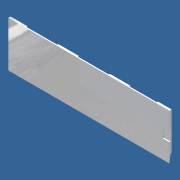
# Autodesk Inventor part: bottom panel left
Saved by Autodesk Inventor 2012 (Build 160160000, 160)
## iProperties
Created: 2012-02-06
Part Number: bottom panel left
Material: Default
Document SubType Name: Modeling
Designer: Allison Garza
Density: 1 g/cm^3
Author: Allison Garza
Autodesk Inventor part; units mm, degrees
ref_plane "YZ Plane" through (0, 0, 0) normal (1, 0, 0) x (0, 1, 0)
ref_plane "XZ Plane" through (0, 0, 0) normal (0, 1, 0) x (-1, 0, 0)
ref_plane "XY Plane" through (0, 0, 0) normal (0, 0, 1) x (1, 0, 0)
sketch "Sketch1" plane through (0, 0, 0) normal (0, 0, 1) x (1, 0, 0)
  line L0 (-37.1429, 20.9244) -> (432.7571, 20.9244)
  line L1 (432.7571, 20.9244) -> (432.7571, -112.4256)
  line L2 (432.7571, -112.4256) -> (-37.1429, -112.4256)
  line L3 (-37.1429, -112.4256) -> (-37.1429, 20.9244)
  point P0 (0, 0)
  dimension "d0" = 469.9
  dimension "d1" = 133.35
  constraints: 8 end point, 2 parallel, 1 horizontal, 1 perpendicular
  measures "d0" distance of L0.start L0.end
  measures "d1" distance of L2.end L0.start
extrude "Extrusion1" add sketch "Sketch1" along normal blind 3.175
sketch "Sketch2" plane through (432.7571, -112.4256, 0) normal (1, 0, 0) x (0, 0, -1)
  line L0 (0, 133.35) -> (0, 0) projected
  line L1 (-3.175, 133.35) -> (0, 107.95)
  line L2 (-3.175, 0) -> (0, 22.86)
  line L3 (-3.175, 0) -> (0, 0)
  line L4 (0, 22.86) -> (0, 0)
  point P0 (0, 112.4256)
  dimension "d4" = 25.4
  dimension "d5" = 22.86
  constraints: 8 end point, 2 perpendicular, 2 point on line
  measures "d4" vertical distance of L1.start L1.end
  measures "d5" vertical distance of L2.end L2.start
extrude "Extrusion3" cut sketch "Sketch2" against normal blind 476.25
sketch "Sketch4" plane through (0, 0, 0) normal (0, 0, -1) x (-1, 0, 0)
  line L0 (-432.7571, -89.5656) -> (37.1429, -89.5656) projected
  line L1 (37.1429, 20.9244) -> (-432.7571, 20.9244) projected
  line L2 (-432.7571, 20.9244) -> (-432.7571, -89.5656) projected
  line L3 (-432.7571, -89.5656) -> (37.1429, -89.5656)
  line L4 (37.1429, -89.5656) -> (37.1429, 20.9244)
  line L5 (37.1429, 20.9244) -> (-432.7571, 20.9244)
  line L6 (-432.7571, 20.9244) -> (-432.7571, -89.5656)
  line L7 (-282.4653, -89.5656) -> (-282.4653, 20.9244)
  line L8 (-132.1735, -89.5656) -> (-132.1735, 20.9244)
  line L9 (18.1183, -89.5656) -> (18.1183, 20.9244)
  line L10 (-282.4653, -89.5656) -> (-312.071, 20.9244)
  line L11 (-432.7571, -89.5656) -> (-392.5421, 20.9244)
  line L12 (-282.4653, -89.5656) -> (-252.8596, 20.9244)
  line L13 (-132.1735, -89.5656) -> (-161.7792, 20.9244)
  line L14 (-132.1735, -89.5656) -> (-102.5678, 20.9244)
  line L15 (18.1183, -89.5656) -> (-11.4874, 20.9244)
  line L16 (18.1183, 20.9244) -> (37.1429, 20.9244)
  line L17 (37.1429, 20.9244) -> (37.1429, -89.5656)
  line L18 (37.1429, -89.5656) -> (18.1183, -89.5656)
  line L19 (18.1183, -89.5656) -> (18.1183, 20.9244)
  point P0 (0, 0)
  dimension "d10" = 150.2918
  dimension "d11" = 150.2918
  dimension "d12" = 150.2918
  dimension "d13" = 20
  dimension "d14" = 15
  dimension "d15" = 15
  constraints: 32 end point, 6 parallel, 5 perpendicular, 3 horizontal, 3 point on line, 12 other
  measures "d10" distance of L0.start L7.start
  measures "d11" distance of L7.start L8.start
  measures "d12" distance of L8.start L9.start
  measures "d13" angle of L2 L11
  measures "d14" angle of L7 L10
  measures "d15" angle of L7 L12
extrude "Extrusion4" add sketch "Sketch4" along normal blind 3.175 contours L2 L1 L11 | L10 L1 L7 | L7 L1 L12 | L13 L1 L8 | L8 L1 L14 | L15 L1 L9
sketch "Sketch5" plane through (0, 0, 0) normal (0, 0, -1) x (-1, 0, 0)
  line L0 (18.1183, 20.9244) -> (18.1183, -89.5656) projected
  line L1 (18.1183, -89.5656) -> (37.1429, -89.5656) projected
  line L2 (37.1429, -89.5656) -> (37.1429, 20.9244) projected
  line L3 (37.1429, 20.9244) -> (18.1183, 20.9244) projected
  line L4 (18.1183, 20.9244) -> (37.1429, 20.9244)
  line L5 (37.1429, 20.9244) -> (37.1429, -89.5656)
  line L6 (37.1429, -89.5656) -> (18.1183, -89.5656)
  line L7 (18.1183, -89.5656) -> (18.1183, 20.9244)
  point P0 (0, 0)
  constraints: 8 end point, 2 parallel, 1 horizontal, 1 perpendicular
sketch "Sketch6" plane through (0, 0, 3.175) normal (0, 0, 1) x (1, 0, 0)
  line L0 (-37.1429, 20.9244) -> (-18.1183, 20.9244)
  line L1 (-18.1183, 20.9244) -> (-18.1183, -89.5656)
  line L2 (-18.1183, -89.5656) -> (-37.1429, -89.5656)
  line L3 (-37.1429, -89.5656) -> (-37.1429, 20.9244)
  point P0 (0, 0)
  dimension "d18" = 110.49
  dimension "d19" = 19.0246
  constraints: 8 end point, 2 parallel, 1 horizontal, 1 perpendicular
  measures "d18" distance of L2.end L0.start
  measures "d19" distance of L1.end L2.end
extrude "Extrusion5" add sketch "Sketch6" against normal blind 6.35
sketch "Sketch9" plane through (0, 0, 3.175) normal (0, 0, 1) x (1, 0, 0)
  line L0 (432.7571, 20.9244) -> (432.7571, -112.4256) projected
  line L1 (432.7571, -33.0506) -> (413.7071, -33.0506)
  line L2 (413.7071, -33.0506) -> (413.7071, -58.4506)
  line L3 (413.7071, -58.4506) -> (432.7571, -58.4506)
  line L4 (432.7571, -58.4506) -> (432.7571, -33.0506)
  point P0 (0, 0)
  dimension "d38" = 25.4
  dimension "d39" = 19.05
  dimension "d40" = 53.975
  constraints: 8 end point, 2 parallel, 1 horizontal, 1 perpendicular, 1 point on line
  measures "d38" distance of L3.end L1.start
  measures "d39" distance of L1.start L1.end
  measures "d40" distance of L0.start L1.start
extrude "Extrusion8" cut sketch "Sketch9" against normal blind 3.175
sketch "Sketch10" plane through (0, 0, 0) normal (0, 0, 1) x (1, 0, 0)
  line L0 (413.7071, -37.2262) -> (421.4322, -58.4506) projected
  line L1 (432.7571, -33.0506) -> (413.7071, -33.0506) projected
  line L2 (413.7071, -33.0506) -> (413.7071, -37.2262) projected
  line L3 (413.7071, -37.2262) -> (421.4322, -58.4506)
  line L4 (413.7071, -58.4506) -> (413.7071, -37.2262)
  line L5 (421.4322, -58.4506) -> (413.7071, -58.4506)
  circle A0 centre (420.0571, -39.4006) radius 1.5875
  circle A1 centre (420.0571, -52.1006) radius 1.5875
  point P0 (0, 0)
  dimension "d43" = 12.7
  dimension "d44" = 6.35
  dimension "d45" = 3.175
  dimension "d46" = 3.175
  dimension "d47" = 6.35
  constraints: 6 end point, 2 centre point, 2 collinear, 1 perpendicular, 1 vertical alignment
  measures "d43" distance of A1.centre A0.centre
  measures "d44" distance from line of L1 A0.centre
  measures "d45" diameter of A0
  measures "d46" diameter of A1
  measures "d47" distance from line of A0.centre L2
extrude "Extrusion9" add sketch "Sketch10" against normal blind 3.175 contours L0 A1 L5 L4 | L0 A1 picked at (419.0163, -52.1007)
extrude "Extrusion10" cut sketch "Sketch10" against normal blind 3.175 contours A1 L0 | L0 A1 | A0
body "Solid1"
